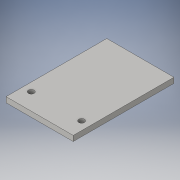
# Autodesk Inventor part: IMUMount
Saved by Autodesk Inventor 2016 (Build 200138000, 138)
## iProperties
Created: 2015-11-13
Part Number: IMUMount
Material: Generic
Document SubType Name: Modeling
Designer: Mack
Density: 1 g/cm^3
Appearance: Default
Author: Mack
Autodesk Inventor part; units mm, degrees
ref_plane "YZ Plane" through (0, 0, 0) normal (1, 0, 0) x (0, 1, 0)
ref_plane "XZ Plane" through (0, 0, 0) normal (0, 1, 0) x (-1, 0, 0)
ref_plane "XY Plane" through (0, 0, 0) normal (0, 0, 1) x (1, 0, 0)
sketch "Sketch1" plane through (0, 0, 0) normal (0, 1, 0) x (-1, 0, 0)
  line L0 (25.4, 38.1) -> (-25.4, 38.1)
  line L1 (-25.4, 38.1) -> (-25.4, -38.1)
  line L2 (-25.4, -38.1) -> (25.4, -38.1)
  line L3 (25.4, -38.1) -> (25.4, 38.1)
  point P0 (0, 0)
  dimension "d0" = 76.2
  dimension "d1" = 50.8
  dimension "d2" = 25.4
  dimension "d3" = 38.1
  constraints: 8 end point, 2 parallel, 1 horizontal, 1 perpendicular
  measures "d0" distance of L2.end L0.start
  measures "d1" distance of L0.start L0.end
  measures "d2" distance from line of point (0, 0) L3
  measures "d3" distance from line of L0 point (0, 0)
extrude "Extrusion1" add sketch "Sketch1" along normal blind 4
sketch "Sketch2" plane through (0, 4, 0) normal (0, 1, 0) x (1, 0, 0)
  line L0 (-25.4, -38.1) -> (25.4, -38.1) projected
  line L1 (-25.4, 38.1) -> (-25.4, -38.1) projected
  point P0 (0, 0)
  point P1 (-19.05, -25.4)
  point P2 (19.05, -25.4)
  dimension "d6" = 12.7
  dimension "d7" = 12.7
  dimension "d8" = 38.1
  dimension "d9" = 6.35
  measures "d6" distance from line of L0 point (-19.05, -25.4)
  measures "d7" distance from line of L0 point (19.05, -25.4)
  measures "d8" distance of point (-19.05, -25.4) point (19.05, -25.4)
  measures "d9" distance from line of L1 point (-19.05, -25.4)
hole "Hole1" at (-19.05, 4, 25.4) at (19.05, 4, 25.4) direction (0, -1, 0) diameter 4.3053 end through all
body "Solid1"
